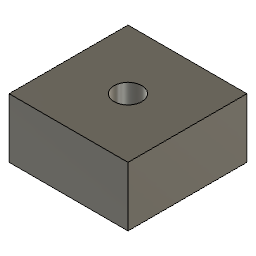
SpacerAbdeckplatte (Autodesk Fusion 360 design; units mm, degrees)
part number: 2025-12-14-22-18-12-909
Autodesk Fusion 360 part; units mm, degrees
sketch "Skizze1" plane through (0, 0, 0) normal (0, 0, 1) x (1, 0, 0)
  line L0 (0, 0) -> (30, 0)
  line L1 (30, 0) -> (30, 30)
  line L2 (30, 30) -> (0, 30)
  line L3 (0, 30) -> (0, 0)
  dimension "d1" = 30
  dimension "d2" = 30
  constraint horizontal L0
  constraint vertical L1
  constraint horizontal L2
  constraint vertical L3
  constraint coincident L0.start L3.end
  measures "d1" distance of L0.start L0.end
  measures "d2" distance of L0.start L2.end
extrude "Extrusion1" add sketch "Skizze1" along normal blind 15
sketch "Skizze2" plane through (0, 0, 15) normal (0, 0, 1) x (-1, 0, 0)
  line L0 (0, -30) -> (0, 0)
  line L1 (0, 0) -> (-30, 0)
  line L2 (-30, 0) -> (-30, -30)
  line L3 (-30, -30) -> (0, -30)
  circle A0 centre (-15, -15) radius 3.5
  dimension "d5" = 7
  measures "d5" diameter of A0
extrude "Extrusion2" cut sketch "Skizze2" against normal blind 15 contours A0
